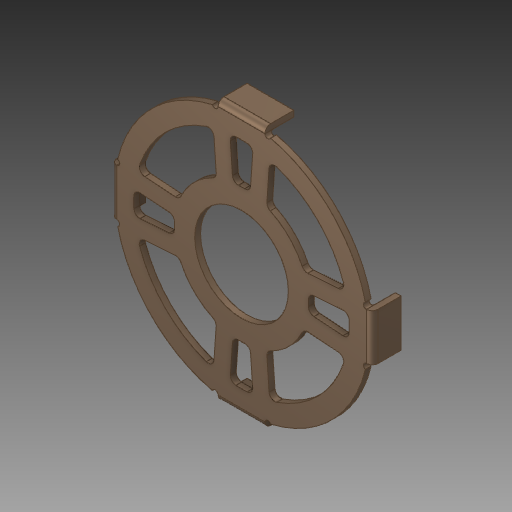
# Autodesk Inventor part: SŁONECZKO
Saved by Autodesk Inventor 2017 SP1 (Build 210196100, 196)
## iProperties
Created: 2021-01-06
Part Number: SŁONECZKO
Material: Stal
Document SubType Name: Modeling
Designer: Napoleon
Mass: 0.94406 g
Surface Area: 5.96996 cm^2
Volume: 0.120262 cm^3
Density: 7.85 g/cm^3
Appearance: Anodowany - brązowy
Author: Napoleon
Autodesk Inventor part; units mm, degrees
ref_plane "YZ Plane" through (0, 0, 0) normal (1, 0, 0) x (0, 1, 0)
ref_plane "XZ Plane" through (0, 0, 0) normal (0, 1, 0) x (-1, 0, 0)
ref_plane "XY Plane" through (0, 0, 0) normal (0, 0, 1) x (1, 0, 0)
sketch "Szkic1" plane through (0, 0, 0) normal (0, 0, 1) x (1, 0, 0)
  circle A0 centre (0, 0) radius 4.05
  line L0 (-11.3, 2.025) -> (-11.3, -2.025)
  line L1 (-10.8, 2.025) -> (-11.3, 2.025)
  line L2 (-9.2716, 0.9962) -> (-5.7517, 0.7466)
  line L3 (-9.0036, 2.4272) -> (-5.3787, 2.1701)
  line L4 (-9.2716, 0.9962) -> (-5.8, 0.75)
  line L5 (-9.2716, -0.9962) -> (-5.7517, -0.7466)
  line L6 (-9.0036, -2.4272) -> (-5.3787, -2.1701)
  line L7 (-9.2716, -0.9962) -> (-5.8, -0.75)
  line L8 (-2.4272, -9.0036) -> (-2.1701, -5.3787)
  line L9 (-0.9962, -9.2716) -> (-0.7466, -5.7517)
  line L10 (-0.9962, -9.2716) -> (-0.75, -5.8)
  line L11 (0.9962, -9.2716) -> (0.7466, -5.7517)
  line L12 (0.9962, -9.2716) -> (0.75, -5.8)
  line L13 (2.4272, -9.0036) -> (2.1701, -5.3787)
  line L14 (9.0036, -2.4272) -> (5.3787, -2.1701)
  line L15 (9.2716, -0.9962) -> (5.7517, -0.7466)
  line L16 (9.2716, -0.9962) -> (5.8, -0.75)
  line L17 (9.2716, 0.9962) -> (5.7517, 0.7466)
  line L18 (9.2716, 0.9962) -> (5.8, 0.75)
  line L19 (9.0036, 2.4272) -> (5.3787, 2.1701)
  line L20 (2.4272, 9.0036) -> (2.1701, 5.3787)
  line L21 (0.9962, 9.2716) -> (0.7466, 5.7517)
  line L22 (0.9962, 9.2716) -> (0.75, 5.8)
  line L23 (-0.9962, 9.2716) -> (-0.7466, 5.7517)
  line L24 (-0.9962, 9.2716) -> (-0.75, 5.8)
  line L25 (-2.4272, 9.0036) -> (-2.1701, 5.3787)
  arc A1 (0.9962, 9.2716) -> (-0.9962, 9.2716) centre (0, 0) ccw
  arc A2 (0.7466, 5.7517) -> (-0.7466, 5.7517) centre (0, 0) ccw
  arc A3 (5.3787, 2.1701) -> (2.1701, 5.3787) centre (0, 0) ccw
  arc A4 (9.0036, 2.4272) -> (2.4272, 9.0036) centre (0, 0) ccw
  arc A5 (9.2716, -0.9962) -> (9.2716, 0.9962) centre (0, 0) ccw
  arc A6 (5.7517, -0.7466) -> (5.7517, 0.7466) centre (0, 0) ccw
  arc A7 (2.4272, -9.0036) -> (9.0036, -2.4272) centre (0, 0) ccw
  arc A8 (2.1701, -5.3787) -> (5.3787, -2.1701) centre (0, 0) ccw
  arc A9 (-0.7466, -5.7517) -> (0.7466, -5.7517) centre (0, 0) ccw
  arc A10 (-0.9962, -9.2716) -> (0.9962, -9.2716) centre (0, 0) ccw
  arc A11 (-9.0036, -2.4272) -> (-2.4272, -9.0036) centre (0, 0) ccw
  arc A12 (-5.3787, -2.1701) -> (-2.1701, -5.3787) centre (0, 0) ccw
  arc A13 (-2.1701, 5.3787) -> (-5.3787, 2.1701) centre (0, 0) ccw
  arc A14 (-5.7517, 0.7466) -> (-5.7517, -0.7466) centre (0, 0) ccw
  arc A15 (-2.4272, 9.0036) -> (-9.0036, 2.4272) centre (0, 0) ccw
  arc A16 (-9.2716, 0.9962) -> (-9.2716, -0.9962) centre (0, 0) ccw
  arc A17 (-10.8, 2.025) -> (-10.7087, 2.5166) centre (-10.8, 2.2793) ccw
  line L26 (-10.8, -2.025) -> (-11.3, -2.025)
  arc A18 (-10.7087, -2.5166) -> (-10.8, -2.025) centre (-10.8, -2.2793) ccw
  line L27 (-2.025, -11.3) -> (2.025, -11.3)
  line L28 (-2.025, -10.8) -> (-2.025, -11.3)
  arc A19 (-2.025, -10.8) -> (-2.5166, -10.7087) centre (-2.2793, -10.8) ccw
  line L29 (2.025, -10.8) -> (2.025, -11.3)
  arc A20 (2.5166, -10.7087) -> (2.025, -10.8) centre (2.2793, -10.8) ccw
  line L30 (11.3, -2.025) -> (11.3, 2.025)
  line L31 (10.8, -2.025) -> (11.3, -2.025)
  arc A21 (10.8, -2.025) -> (10.7087, -2.5166) centre (10.8, -2.2793) ccw
  line L32 (10.8, 2.025) -> (11.3, 2.025)
  arc A22 (10.7087, 2.5166) -> (10.8, 2.025) centre (10.8, 2.2793) ccw
  line L33 (2.025, 11.3) -> (-2.025, 11.3)
  line L34 (2.025, 10.8) -> (2.025, 11.3)
  arc A23 (2.025, 10.8) -> (2.5166, 10.7087) centre (2.2793, 10.8) ccw
  line L35 (-2.025, 10.8) -> (-2.025, 11.3)
  arc A24 (-2.5166, 10.7087) -> (-2.025, 10.8) centre (-2.2793, 10.8) ccw
  arc A25 (-10.7083, -2.5164) -> (-2.5164, -10.7083) centre (0, 0) ccw
  arc A26 (2.5164, -10.7083) -> (10.7083, -2.5164) centre (0, 0) ccw
  arc A27 (-2.5164, 10.7083) -> (-10.7083, 2.5164) centre (0, 0) ccw
  arc A28 (10.7083, 2.5164) -> (2.5164, 10.7083) centre (0, 0) ccw
  dimension "d19" = 360
  dimension "d28" = 360
  constraints: 72 end point, 64 point on circle, 29 centre point, 3 coincident, 1 tangent, 118 other
extrude "Wyciągnięcie proste1" add sketch "Szkic1" against normal blind 0.5
fillet "Zaokrąglenie1" radius 0.5 32 edges at (-9.2716, 0.9962, -0.25) (-5.7517, 0.7466, -0.25) (-5.7517, -0.7466, -0.25) (-9.2716, -0.9962, -0.25) (-9.0036, 2.4272, -0.25) (-5.3787, 2.1701, -0.25) (-2.1701, 5.3787, -0.25) (-2.4272, 9.0036, -0.25) (-0.9962, 9.2716, -0.25) (-0.7466, 5.7517, -0.25) (0.7466, 5.7517, -0.25) (0.9962, 9.2716, -0.25) (2.4272, 9.0036, -0.25) (2.1701, 5.3787, -0.25) (5.3787, 2.1701, -0.25) (9.0036, 2.4272, -0.25) (5.7517, 0.7466, -0.25) (5.7517, -0.7466, -0.25) (9.2716, -0.9962, -0.25) (9.2716, 0.9962, -0.25) (5.3787, -2.1701, -0.25) (9.0036, -2.4272, -0.25) (2.1701, -5.3787, -0.25) (2.4272, -9.0036, -0.25) (-0.7466, -5.7517, -0.25) (0.7466, -5.7517, -0.25) (0.9962, -9.2716, -0.25) (-0.9962, -9.2716, -0.25) (-2.1701, -5.3787, -0.25) (-2.4272, -9.0036, -0.25) (-9.0036, -2.4272, -0.25) (-5.3787, -2.1701, -0.25)
sketch "Szkic2" plane through (0, 0, -0.5) normal (0, 0, -1) x (-1, 0, 0)
  arc A0 (-10.7083, -2.5164) -> (-10.8, -2.025) centre (-10.8, -2.2793) ccw projected
  line L0 (-11.3, 2.025) -> (-10.8, 2.025) projected
  line L1 (-11.3, 2.025) -> (-10.8, 2.025)
  line L2 (-10.8, 2.025) -> (-10.8, -2.025)
  line L3 (-10.8, -2.025) -> (-11.3, -2.025)
  line L4 (-11.3, -2.025) -> (-11.3, 2.025)
  line L5 (-2.025, 11.3) -> (2.025, 11.3)
  line L6 (2.025, 11.3) -> (2.025, 10.8)
  line L7 (2.025, 10.8) -> (-2.025, 10.8)
  line L8 (-2.025, 10.8) -> (-2.025, 11.3)
  line L9 (11.3, 2.025) -> (10.8, 2.025)
  line L10 (10.8, 2.025) -> (10.8, -2.025)
  line L11 (10.8, -2.025) -> (11.3, -2.025)
  line L12 (11.3, -2.025) -> (11.3, 2.025)
  line L13 (-2.025, -11.3) -> (2.025, -11.3)
  line L14 (2.025, -11.3) -> (2.025, -10.8)
  line L15 (2.025, -10.8) -> (-2.025, -10.8)
  line L16 (-2.025, -10.8) -> (-2.025, -11.3)
  constraints: 32 end point, 8 parallel, 4 horizontal, 4 perpendicular, 1 point on circle
extrude "Wyciągnięcie proste2" add sketch "Szkic2" along normal blind 2
fillet "Zaokrąglenie2" radius 0.5 4 edges at (0, 11.3, 0) (11.3, 0, 0) (0, -11.3, 0) (-11.3, 0, 0)
fillet "Zaokrąglenie3" radius 0.25 4 edges at (0, -10.8, -0.5) (-10.8, 0, -0.5) (10.8, 0, -0.5) (0, 10.8, -0.5)
